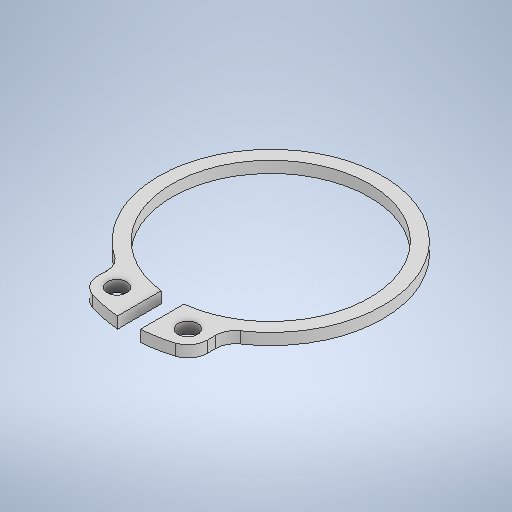
# Autodesk Inventor part: 49-01-003
Saved by Autodesk Inventor 2025.2 (Build 292293000, 293)
## iProperties
Created: 2024-11-28
Part Number: 49-01-003
Material: Generic
Document SubType Name: Modeling
Designer: Zvonko.Gabric
Density: 1 g/cm^3
Appearance: Default
Author: Zvonko.Gabric
Autodesk Inventor part; units mm, degrees
ref_plane "YZ Plane" through (0, 0, 0) normal (1, 0, 0) x (0, 1, 0)
ref_plane "XZ Plane" through (0, 0, 0) normal (0, 1, 0) x (-1, 0, 0)
ref_plane "XY Plane" through (0, 0, 0) normal (0, 0, 1) x (1, 0, 0)
sketch "Sketch1" plane through (0, 0, 0) normal (0, 1, 0) x (-1, 0, 0)
  line L0 (5.1326, 19.4481) -> (5.1326, 20.2053)
  line L1 (14.7968, 20.1543) -> (14.7968, 19.3971)
  line L2 (10.897, 18.4868) -> (10.897, 22.3047)
  line L3 (8.8887, 22.3071) -> (8.8887, 18.4892)
  circle A0 centre (13.0968, 20.1543) radius 0.85
  circle A1 centre (6.8326, 20.2053) radius 0.85
  arc A2 (4.384, 18.0392) -> (5.1326, 19.4481) centre (3.4326, 19.4481) ccw
  arc A3 (4.384, 18.0392) -> (15.3812, 18.0392) centre (9.8826, 9.897) ccw
  arc A4 (14.7968, 19.3971) -> (15.3812, 18.0392) centre (16.4952, 19.3234) ccw
  arc A5 (14.7968, 20.1543) -> (13.6051, 21.7765) centre (13.0968, 20.1543) ccw
  arc A6 (13.6051, 21.7765) -> (10.897, 22.3047) centre (9.8826, 9.897) ccw
  arc A7 (8.8887, 18.4892) -> (10.897, 18.4868) centre (9.8826, 9.897) ccw
  arc A8 (8.8887, 22.3071) -> (6.3243, 21.8275) centre (9.8826, 9.897) ccw
  arc A9 (6.3243, 21.8275) -> (5.1326, 20.2053) centre (6.8326, 20.2053) ccw
  point P0 (0, 0)
  dimension "d0" = 0
  dimension "d1" = 0
  dimension "d2" = 0
  dimension "d5" = 8.6495
  dimension "d6" = 9.825
  dimension "d7" = 1.7
  dimension "d8" = 1.7
  dimension "d9" = 1.7
  dimension "d10" = 1.7
  dimension "d11" = 6.2642
  dimension "d12" = 2.0084
  dimension "d13" = 1.7
  dimension "d14" = 1.7
  dimension "d15" = 12.4491
  dimension "d16" = 12.4499
  constraints: 16 point on circle, 10 centre point, 8 end point
  measures "d0" distance of A1.centre A9.centre
  measures "d1" distance of A0.centre A5.centre
  measures "d2" distance of A3.centre A6.centre
  measures "d5" radius of A7
  measures "d6" radius of A3
  measures "d7" radius of A4
  measures "d8" radius of A2
  measures "d9" diameter of A1
  measures "d10" diameter of A0
  measures "d11" horizontal distance of A0.centre A1.centre
  measures "d12" distance between parallel lines of L2 L3
  measures "d13" radius of A5
  measures "d14" radius of A9
  measures "d15" radius of A6
  measures "d16" radius of A8
extrude "Extrusion1" add sketch "Sketch1" along normal blind 1
body "Solid1"
